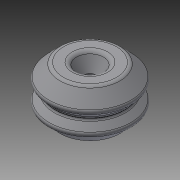
# Autodesk Inventor part: VertebraeSimple2
Saved by Autodesk Inventor 2014 SP1 (Build 180222100, 222)
## iProperties
Created: 2014-11-10
Part Number: VertebraeSimple2
Material: Generic
Document SubType Name: Modeling
Designer: rawrdong
Density: 1 g/cm^3
Appearance: Default
Author: rawrdong
Autodesk Inventor part; units mm, degrees
ref_plane "YZ Plane" through (0, 0, 0) normal (1, 0, 0) x (0, 1, 0)
ref_plane "XZ Plane" through (0, 0, 0) normal (0, 1, 0) x (-1, 0, 0)
ref_plane "XY Plane" through (0, 0, 0) normal (0, 0, 1) x (1, 0, 0)
sketch "Sketch1" plane through (0, 0, 0) normal (1, 0, 0) x (0, 1, 0)
  line L0 (-4.4429, 0) -> (26.6577, 0) projected
  line L1 (0, 15.6393) -> (0, -6.3359) construction
  line L2 (3.375, 0) -> (3.375, -3.1966) construction
  line L3 (3.375, 5) -> (7.7051, 12.5)
  line L4 (7.7051, 12.5) -> (14.7147, 12.5)
  line L5 (14.7147, 12.5) -> (22.2147, 5)
  line L6 (22.2147, 5) -> (17.8777, 0.663)
  line L7 (17.8777, 0.663) -> (17.8777, 0)
  line L8 (3.375, 5) -> (3.375, 0)
  line L9 (3.375, 0) -> (17.8777, 0)
  point P0 (0, 0)
  dimension "d0" = 3.375
  dimension "d1" = 45
  dimension "d2" = 30
  dimension "d3" = 45
  dimension "d8" = 12.5
  dimension "d11" = 5
  constraints: 16 end point, 3 point on line, 2 collinear, 2 perpendicular, 1 horizontal alignment, 1 parallel
  measures "d0" distance between parallel lines of L1 L2
  measures "d1" angle of L0 L5
  measures "d2" angle of L2 L3
  measures "d3" angle of L6 L0
  measures "d8" distance between parallel lines of L0 L4
  measures "d11" distance of L3.start L2.start
revolve "Revolution1" add sketch "Sketch1" angle 360 about axis through (0, 0, 0) along (0, 0, -1)
mirror "Mirror1" about plane through (0, 3.375, 0) normal (0, 0, -1) of "Revolution1"
fillet "Fillet1" radius 1.5 4 edges at (0, -22.2147, 5) (0, -22.2147, -5) (0, -17.8777, 0.663) (0, -17.8777, -0.663)
fillet "Fillet2" radius 2.5 4 edges at (0, -7.7051, 12.5) (0, -14.7147, 12.5) (0, -7.7051, -12.5) (0, -14.7147, -12.5)
body "Solid1"
